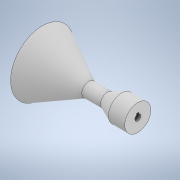
# Autodesk Inventor part: SpacerA
Saved by Autodesk Inventor 2021.2 (Build 252289000, 289)
## iProperties
Created: 2021-05-18
Part Number: SpacerA
Material: Generic
Document SubType Name: Modeling
Designer: Ryan
Density: 1 g/cm^3
Appearance: Default
Author: Ryan
Autodesk Inventor part; units mm, degrees
ref_plane "YZ Plane" through (0, 0, 0) normal (1, 0, 0) x (0, 1, 0)
ref_plane "XZ Plane" through (0, 0, 0) normal (0, 1, 0) x (-1, 0, 0)
ref_plane "XY Plane" through (0, 0, 0) normal (0, 0, 1) x (1, 0, 0)
sketch "Sketch1" plane through (0, 0, 0) normal (0, 0, 1) x (1, 0, 0)
  line L0 (0, 0) -> (0, 43.18)
  line L1 (0, 43.18) -> (63.5, 9.525)
  line L2 (88.9, 9.525) -> (107.95, 17.78)
  line L3 (107.95, 17.78) -> (130.175, 17.78)
  line L4 (130.175, 17.78) -> (130.175, 0)
  line L5 (0, 0) -> (130.175, 0)
  line L6 (63.5, 9.525) -> (88.9, 9.525)
  line L7 (0, 4) -> (130.175, 4)
  dimension "d0" = 43.18
  dimension "d6" = 22.225
  dimension "d14" = 4
  dimension "d17" = 9.525
  dimension "d18" = 17.78
  dimension "d21" = 25.4
  dimension "d22" = 63.5
  dimension "d29" = 19.05
  constraints: 16 end point, 3 perpendicular, 2 point on line, 1 horizontal, 1 vertical
  measures "d0" distance of L0.start L0.end
  measures "d6" distance of L2.end L3.end
  measures "d14" distance between parallel lines of L5 L7
  measures "d17" distance between parallel lines of L5 L6
  measures "d18" distance of L3.end L4.end
  measures "d21" distance of L1.end L2.start
  measures "d22" distance from line of L0 L1.end
  measures "d29" horizontal distance of L2.end L2.start
revolve "Revolution1" add sketch "Sketch1" angle 360 about axis through (0, 0, 0) along (1, 0, 0) contours L0 L1 L6 L2 L3 L4 L7
sketch "Sketch2" plane through (0, 0, 0) normal (-1, 0, 0) x (0, 0, 1)
  line L0 (-1.5875, 5.5875) -> (1.5875, 5.5875)
  line L1 (1.5875, 5.5875) -> (1.5875, 2.4125)
  line L2 (1.5875, 2.4125) -> (-1.5875, 2.4125)
  line L3 (-1.5875, 2.4125) -> (-1.5875, 5.5875)
  circle A0 centre (0, 0) radius 4 projected
  line L4 (-1.5875, 5.5875) -> (1.5875, 2.4125) construction
  line L5 (1.5875, 5.5875) -> (-1.5875, 2.4125) construction
  point P0 (0, 4)
  dimension "d24" = 3.175
  dimension "d25" = 3.175
  constraints: 12 end point, 2 midpoint, 2 parallel, 1 horizontal, 1 perpendicular, 1 vertical alignment, 1 other
  measures "d24" distance of L1.end L2.end
  measures "d25" distance of L0.end L1.end
extrude "Extrusion1" cut sketch "Sketch2" against normal through all contours L0 L1 A0 L3 | A0 L1 L2 L3 picked at (0, 2.9417)
body "Solid1"
